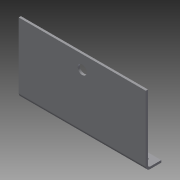
# Autodesk Inventor part: Front wheel mount plate
Saved by Autodesk Inventor 2014 (Build 180170000, 170)
## iProperties
Created: 2014-02-17
Part Number: Front wheel mount plate
Material: Generic
Document SubType Name: Sheet Metal
Designer: Michael
Density: 1 g/cm^3
Sheet Metal Rule: Default
Appearance: Default
Flat Pattern Width: 11.43 cm
Flat Pattern Length: 17.78 cm
Flat Pattern Area: 203.225 cm^2
Sheet Metal Width: 4.500 in
Sheet Metal Length: 7.000 in
Sheet Metal Area: 31.500 in^2
Author: Michael
Autodesk Inventor part; units mm, degrees
ref_plane "YZ Plane" through (0, 0, 0) normal (1, 0, 0) x (0, 1, 0)
ref_plane "XZ Plane" through (0, 0, 0) normal (0, 1, 0) x (-1, 0, 0)
ref_plane "XY Plane" through (0, 0, 0) normal (0, 0, 1) x (1, 0, 0)
sketch "Sketch1" plane through (0, 0, 0) normal (0, 0, 1) x (1, 0, 0)
  line L0 (0, 0) -> (177.8, 0)
  line L1 (177.8, 0) -> (177.8, 114.3)
  line L2 (177.8, 114.3) -> (0, 114.3)
  line L3 (0, 114.3) -> (0, 0)
  line L4 (0, 0) -> (0, 9.525) construction
  line L5 (0, 9.525) -> (12.7, 9.525) construction
  line L6 (177.8, 0) -> (177.8, 9.525) construction
  line L7 (177.8, 9.525) -> (165.1, 9.525) construction
  circle A0 centre (12.7, 9.525) radius 3.175
  circle A1 centre (165.1, 9.525) radius 3.175
  circle A2 centre (88.9, 95.25) radius 6.35
  line L8 (0, 0) -> (0, 19.05) construction
  line L9 (0, 19.05) -> (177.8, 19.05)
  dimension "d0" = 177.8
  dimension "d1" = 114.3
  dimension "d2" = 9.525
  dimension "d3" = 12.7
  dimension "d4" = 9.525
  dimension "d5" = 12.7
  dimension "d7" = 6.35
  dimension "d8" = 6.35
  dimension "d9" = 12.7
  dimension "d10" = 19.05
  dimension "d11" = 76.2
  constraints: 20 end point, 4 perpendicular, 4 point on line, 3 centre point, 2 coincident, 2 parallel, 1 horizontal
  measures "d0" distance of L2.end L1.end
  measures "d1" distance of L1.end L0.end
  measures "d2" distance of L0.start L4.end
  measures "d3" distance of L4.end L5.end
  measures "d4" distance of L0.end L6.end
  measures "d5" distance of L6.end L7.end
  measures "d7" diameter of A0
  measures "d8" diameter of A1
  measures "d9" diameter of A2
  measures "d10" distance of L0.start L8.end
  measures "d11" distance from line of L9 A2.centre
extrude "Plate1" add sketch "Sketch1" along normal blind 3.048
fold "Fold1" angle 90 bend radius 3.048 thickness 3.048 k factor 0.44 line from (0, 19.05, 0) to (177.8, 19.05, 0) line at bend centre moving side (0, -1, 0) folds toward (0, 0, -1)
equation "\"d13\" = BendReliefWidth"
equation "\"d14\" = BendReliefDepth"
equation "\"d15\" = MinimumRemnant"
equation "\"d16\" = BendRadius"
equation "\"d18\" = BendRadius"
equation "\"BendRadius\" = Thickness"
equation "\"BendReliefWidth\" = Thickness"
equation "\"BendReliefDepth\" = 0.5 * Thickness"
equation "\"CornerReliefSize\" = 4 * Thickness"
equation "\"MinimumRemnant\" = 2 * Thickness"
equation "\"TransitionRadius\" = BendRadius"
equation "\"JacobiRadiusSize\" = BendRadius"
equation "\"GapSize\" = Thickness"
equation "\"d12\" = BendRadius"
equation "\"Thickness\" = 3.048"
body "Solid1"
